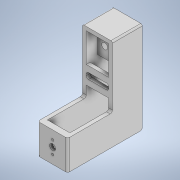
# Autodesk Inventor part: Link4_v2
Saved by Autodesk Inventor 2022 (Build 260153000, 153)
## iProperties
Created: 2022-06-14
Part Number: Link4_v2
Material: Generic
Document SubType Name: Modeling
Designer: Asus
Density: 1 g/cm^3
Appearance: Default
Author: Asus
Autodesk Inventor part; units mm, degrees
ref_plane "YZ Plane" through (0, 0, 0) normal (1, 0, 0) x (0, 1, 0)
ref_plane "XZ Plane" through (0, 0, 0) normal (0, 1, 0) x (-1, 0, 0)
ref_plane "XY Plane" through (0, 0, 0) normal (0, 0, 1) x (1, 0, 0)
sketch "Sketch1" plane through (0, 0, 0) normal (0, 0, 1) x (1, 0, 0)
  line L0 (-20, 22.5) -> (20, 22.5)
  line L1 (20, 22.5) -> (20, -100)
  line L2 (20, -100) -> (-20, -100)
  line L3 (-20, -100) -> (-20, 22.5)
  circle A0 centre (0, 0) radius 2.5
  dimension "d0" = 122.5
  dimension "d1" = 40
  dimension "d2" = 20
  dimension "d3" = 22.5
  dimension "d4" = 5
  constraints: 8 end point, 2 parallel, 1 centre point, 1 coincident, 1 horizontal, 1 perpendicular
  measures "d0" distance of L0.end L1.end
  measures "d1" distance of L0.start L0.end
  measures "d2" distance from line of point (0, 0) L1
  measures "d3" distance from line of L0 point (0, 0)
  measures "d4" diameter of A0
extrude "Extrusion1" add sketch "Sketch1" along normal blind 5
sketch "Sketch2" plane through (0, 0, 5) normal (0, 0, 1) x (1, 0, 0)
  line L0 (20, 22.5) -> (-20, 22.5) projected
  line L1 (-20, -100) -> (20, -100) projected
  line L2 (-20, 22.5) -> (20, 22.5)
  line L3 (20, 22.5) -> (20, -100)
  line L4 (20, -100) -> (-20, -100)
  line L5 (-20, -100) -> (-20, 22.5)
  line L6 (15, -95) -> (-15, -95)
  line L7 (-15, -95) -> (-15, 17.5)
  line L8 (-15, 17.5) -> (15, 17.5)
  line L9 (15, 17.5) -> (15, -95)
  point P0 (0, 0)
  dimension "d7" = 5
  dimension "d8" = 5
  dimension "d9" = 5
  dimension "d10" = 5
  constraints: 16 end point, 4 parallel, 2 horizontal, 2 perpendicular
  measures "d7" distance between parallel lines of L0 L8
  measures "d8" distance between parallel lines of L7 L5
  measures "d9" distance between parallel lines of L9 L3
  measures "d10" distance between parallel lines of L6 L1
extrude "Extrusion2" add sketch "Sketch2" along normal blind 35
sketch "Sketch3" plane through (-20, -100, 0) normal (0, -1, 0) x (1, 0, 0)
  circle A0 centre (20, 20) radius 8.5
  line L0 (40, 0) -> (40, 40) projected
  line L1 (0, 0) -> (40, 0) projected
  circle A1 centre (20, 11.5) radius 1.5
  circle A2 centre (20, 28.5) radius 1.5
  circle A3 centre (20, 20) radius 3.75
  line L2 (0, 0) -> (0, 40) projected
  point P0 (20, 0)
  dimension "d13" = 20
  dimension "d14" = 20
  dimension "d15" = 17
  dimension "d16" = 3
  dimension "d17" = 7.5
  dimension "d18" = 3
  dimension "d19" = 20
  dimension "d20" = 20
  constraints: 4 centre point, 2 point on circle, 1 coincident
  measures "d13" distance from line of L0 A0.centre
  measures "d14" distance from line of L1 A0.centre
  measures "d15" diameter of A0
  measures "d16" diameter of A2
  measures "d17" diameter of A3
  measures "d18" diameter of A1
  measures "d19" distance from line of L2 A1.centre
  measures "d20" distance from line of L2 A2.centre
sketch "Sketch4" plane through (0, 0, 5) normal (0, 0, 1) x (1, 0, 0)
  line L0 (-15, 17.5) -> (-15, -95) projected
  line L1 (15, 17.5) -> (15, -95) projected
  line L2 (-15, 17.5) -> (15, 17.5)
  line L3 (15, 17.5) -> (15, -17.5)
  line L4 (15, -17.5) -> (-15, -17.5)
  line L5 (-15, -17.5) -> (-15, 17.5)
  point P0 (0, 0)
  point P1 (-15, -17.5)
  dimension "d21" = 35
  constraints: 8 end point, 2 parallel, 1 horizontal, 1 perpendicular, 1 point on line
  measures "d21" distance between parallel lines of L2 L4
extrude "Extrusion3" add sketch "Sketch4" along normal blind 20
sketch "Sketch5" plane through (0, 0, 0) normal (0, 0, -1) x (-1, 0, 0)
  circle A0 centre (0, 0) radius 2.5 projected
  circle A1 centre (0, 0) radius 9.5
  dimension "d24" = 19
  constraints: 1 centre point, 1 coincident
  measures "d24" diameter of A1
extrude "Extrusion4" cut sketch "Sketch5" against normal blind 12.5 contours A0 | A1
sketch "Sketch6" plane through (0, 0, 0) normal (0, 0, -1) x (-1, 0, 0)
  circle A0 centre (0, 0) radius 11.5
  dimension "d27" = 23
  constraints: 1 centre point, 1 coincident
  measures "d27" diameter of A0
extrude "Extrusion5" cut sketch "Sketch6" against normal blind 6.5
fillet "Fillet1" radius 2 2 edges at (-20, 22.5, 20) (20, 22.5, 20)
sketch "Sketch7" plane through (0, 0, 0) normal (0, 0, -1) x (-1, 0, 0)
  circle A0 centre (0, 0) radius 6.2
  circle A1 centre (0, 6.2) radius 1.45
  line L0 (0, 6.2) -> (0, 0)
  line L1 (0, 0) -> (6.4707, -3.7359)
  line L2 (0, 0) -> (-6.6791, -3.8562)
  circle A2 centre (5.3694, -3.1) radius 1.45
  circle A3 centre (-5.3694, -3.1) radius 1.45
  dimension "d31" = 12.4
  dimension "d32" = 120
  dimension "d33" = 120
  dimension "d34" = 2.9
  dimension "d35" = 2.9
  dimension "d36" = 2.9
  constraints: 6 end point, 4 centre point, 3 point on circle, 2 point on line, 1 coincident, 1 vertical
  measures "d31" diameter of A0
  measures "d32" angle of L0 L2
  measures "d33" angle of L1 L2
  measures "d34" diameter of A1
  measures "d35" diameter of A3
  measures "d36" diameter of A2
extrude "Extrusion6" cut sketch "Sketch7" against normal blind 25 contours A1 L0 A0 | A0 A1 | A2 A0 | A0 L1 A2 | L0 A1 A0 | A0 A2 L1 | A3 L2 A0 | A0 L2 A3 | A3 A0 L2 | A3 L2 A0
sketch "Sketch8" plane through (0, 0, 25) normal (0, 0, 1) x (1, 0, 0)
  circle A0 centre (5.3694, -3.1) radius 1.45 projected
  circle A1 centre (5.3694, -3.1) radius 4
  circle A2 centre (-5.3694, -3.1) radius 1.45 projected
  circle A3 centre (-5.3694, -3.1) radius 4
  circle A4 centre (0, 6.2) radius 1.45 projected
  circle A5 centre (0, 6.2) radius 4
  point P0 (0, 0)
  dimension "d39" = 8
  dimension "d40" = 8
  dimension "d41" = 8
  constraints: 3 centre point, 3 coincident
  measures "d39" diameter of A5
  measures "d40" diameter of A1
  measures "d41" diameter of A3
extrude "Extrusion7" cut sketch "Sketch8" against normal blind 7
fillet "Fillet2" radius 2 3 edges at (0, -17.5, 5) (-15, -56.25, 5) (15, -56.25, 5)
sketch "Sketch9" plane through (0, 0, 40) normal (0, 0, 1) x (1, 0, 0)
  line L0 (20, -100) -> (20, 20.5) projected
  line L1 (-20, 20.5) -> (-20, -100) projected
  line L2 (20, -100) -> (-20, -100)
  line L3 (-20, -100) -> (-20, -60)
  line L4 (-20, -60) -> (20, -60)
  line L5 (20, -60) -> (20, -100)
  line L6 (0, -60) -> (-20, -60)
  line L7 (-20, -60) -> (-20, -100)
  line L8 (-20, -100) -> (0, -100)
  line L9 (0, -100) -> (0, -60)
  line L10 (15, -95) -> (-15, -95) projected
  line L11 (15, -65) -> (-15, -65)
  line L12 (-15, -65) -> (-15, -95)
  line L13 (-15, -95) -> (15, -95)
  line L14 (15, -95) -> (15, -65)
  point P0 (0, 0)
  dimension "d45" = 40
  dimension "d46" = 5
  dimension "d47" = 5
  constraints: 24 end point, 6 parallel, 3 horizontal, 3 perpendicular, 1 midpoint, 1 point on line
  measures "d45" distance between parallel lines of L2 L4
  measures "d46" distance between parallel lines of L0 L14
  measures "d47" distance between parallel lines of L11 L4
extrude "Extrusion8" add sketch "Sketch9" along normal blind 60 contours L2 L9 L10 L14 L11 L4 L0 | L2 L1 L4 L9 L11 L12 L10
sketch "Sketch10" plane through (0, 0, 100) normal (0, 0, 1) x (1, 0, 0)
  line L0 (-20, -100) -> (20, -100) projected
  line L1 (20, -100) -> (20, 20.5) projected
  line L2 (-20, -100) -> (20, -100)
  line L3 (20, -100) -> (20, -60)
  line L4 (20, -60) -> (-20, -60)
  line L5 (-20, -60) -> (-20, -100)
  point P0 (0, 0)
  dimension "d50" = 40
  constraints: 8 end point, 2 parallel, 1 horizontal, 1 perpendicular, 1 point on line
  measures "d50" distance between parallel lines of L0 L4
extrude "Extrusion9" add sketch "Sketch10" against normal blind 5
sketch "Sketch11" plane through (0, 0, 100) normal (0, 0, 1) x (1, 0, 0)
  circle A0 centre (0, -80) radius 8.5
  line L0 (20, -100) -> (20, -60) projected
  line L1 (-20, -100) -> (20, -100) projected
  circle A1 centre (0, -71.5) radius 1.5
  circle A2 centre (0, -88.5) radius 1.5
  line L2 (-20, -60) -> (-20, -100) projected
  circle A3 centre (0, -80) radius 4
  point P0 (0, 0)
  dimension "d53" = 20
  dimension "d54" = 20
  dimension "d55" = 17
  dimension "d56" = 3
  dimension "d57" = 3
  dimension "d58" = 20
  dimension "d59" = 20
  dimension "d62" = 8
  constraints: 4 centre point, 2 point on circle, 1 coincident
  measures "d53" distance from line of L0 A0.centre
  measures "d54" distance from line of L1 A0.centre
  measures "d55" diameter of A0
  measures "d56" diameter of A1
  measures "d57" diameter of A2
  measures "d58" distance from line of L2 A2.centre
  measures "d59" distance from line of L2 A1.centre
  measures "d62" diameter of A3
extrude "Extrusion10" cut sketch "Sketch11" against normal blind 5 contours A1 A0 | A0 A1 | A2 A0 | A0 A2 | A3
sketch "Sketch12" plane through (-15, -60, 40) normal (0, 1, 0) x (1, 0, 0)
  line L0 (0, 0) -> (30, 0) projected
  line L1 (0, 0) -> (30, 0)
  line L2 (30, 0) -> (30, -55)
  line L3 (30, -55) -> (0, -55)
  line L4 (0, -55) -> (0, 0)
  point P0 (15, 40)
  constraints: 8 end point, 2 parallel, 1 horizontal, 1 perpendicular
extrude "Extrusion11" cut sketch "Sketch12" against normal blind 5
sketch "Sketch13" plane through (0, 0, 40) normal (0, 0, 1) x (1, 0, 0)
  line L0 (-20, 20.5) -> (-20, -100) projected
  line L1 (20, -60) -> (20, 20.5) projected
  line L2 (-20, -21.5352) -> (20, -21.5352)
  line L3 (20, -21.5352) -> (20, -29.5352)
  line L4 (20, -29.5352) -> (-20, -29.5352)
  line L5 (-20, -29.5352) -> (-20, -21.5352)
  line L6 (20, -37.5352) -> (-20, -37.5352)
  line L7 (-20, -37.5352) -> (-20, -45.5352)
  line L8 (-20, -45.5352) -> (20, -45.5352)
  line L9 (20, -45.5352) -> (20, -37.5352)
  point P0 (0, 0)
  point P1 (-20, -37.5352)
  point P2 (-20, -29.5352)
  point P3 (20, -21.5352)
  dimension "d65" = 8
  dimension "d66" = 8
  dimension "d67" = 8
  constraints: 16 end point, 4 parallel, 4 point on line, 2 horizontal, 2 perpendicular
  measures "d65" distance between parallel lines of L6 L8
  measures "d66" distance between parallel lines of L2 L4
  measures "d67" distance between parallel lines of L4 L6
extrude "Extrusion12" add sketch "Sketch13" against normal blind 5 contours L2 L1 L4 L0 | L6 L1 L8 L0
fillet "Fillet3" radius 3 4 edges at (15, -29.5352, 37.5) (15, -37.5352, 37.5) (-15, -29.5352, 37.5) (-15, -37.5352, 37.5)
sketch "Sketch14" plane through (0, 0, 95) normal (0, 0, -1) x (-1, 0, 0)
  line L0 (15, -95) -> (-15, -95) projected
  line L1 (-15, -95) -> (15, -95)
  line L2 (15, -95) -> (15, -60)
  line L3 (15, -60) -> (-15, -60)
  line L4 (-15, -60) -> (-15, -95)
  circle A0 centre (0, -80) radius 4 projected
  circle A1 centre (0, -80) radius 4
  circle A2 centre (0, -71.5) radius 1.5 projected
  circle A3 centre (0, -71.5) radius 1.5
  circle A4 centre (0, -88.5) radius 1.5 projected
  circle A5 centre (0, -88.5) radius 1.5
  point P0 (0, 0)
  constraints: 8 end point, 3 centre point, 3 coincident, 2 parallel, 1 horizontal, 1 perpendicular
extrude "Extrusion13" add sketch "Sketch14" along normal blind 3
sketch "Sketch15" plane through (0, 0, 92) normal (0, 0, -1) x (-1, 0, 0)
  circle A0 centre (0, -80) radius 4 projected
  circle A1 centre (0, -80) radius 13
  point P0 (0, 0)
  dimension "d73" = 26
  constraints: 1 centre point, 1 coincident
  measures "d73" diameter of A1
extrude "Extrusion14" cut sketch "Sketch15" against normal blind 4 contours A0 | A1
fillet "Fillet4" radius 3 5 edges at (-20, -80, 100) (20, -80, 100) (-17.5, -60, 40) (17.5, -60, 40) (0, -100, 0)
body "Solid1"
